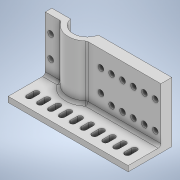
# Autodesk Inventor part: CLAMP2
Saved by Autodesk Inventor 2022 (Build 260153000, 153)
## iProperties
Created: 2022-02-10
Part Number: CLAMP2
Material: Generic
Document SubType Name: Modeling
Designer: 24sa01
Density: 1 g/cm^3
Appearance: Default
Author: 24sa01
Autodesk Inventor part; units mm, degrees
ref_plane "YZ Plane" through (0, 0, 0) normal (1, 0, 0) x (0, 1, 0)
ref_plane "XZ Plane" through (0, 0, 0) normal (0, 1, 0) x (-1, 0, 0)
ref_plane "XY Plane" through (0, 0, 0) normal (0, 0, 1) x (1, 0, 0)
sketch "Sketch1" plane through (0, 0, 0) normal (0, 1, 0) x (-1, 0, 0)
  line L0 (0, 0) -> (-139.7, 0)
  line L1 (-139.7, 0) -> (-139.7, -50.8)
  line L2 (-139.7, -50.8) -> (0, -50.8)
  line L3 (0, -50.8) -> (0, 0)
  line L4 (-12.7, -11.7475) -> (-12.7, -20.0025) construction
  line L5 (-15.875, -11.7475) -> (-15.875, -20.0025)
  line L6 (-9.525, -20.0025) -> (-9.525, -11.7475)
  arc A0 (-9.525, -11.7475) -> (-15.875, -11.7475) centre (-12.7, -11.7475) ccw
  arc A1 (-15.875, -20.0025) -> (-9.525, -20.0025) centre (-12.7, -20.0025) ccw
  line L7 (-25.4, -11.7475) -> (-25.4, -20.0025) construction
  line L8 (-28.575, -11.7475) -> (-28.575, -20.0025)
  line L9 (-22.225, -20.0025) -> (-22.225, -11.7475)
  arc A2 (-22.225, -11.7475) -> (-28.575, -11.7475) centre (-25.4, -11.7475) ccw
  arc A3 (-28.575, -20.0025) -> (-22.225, -20.0025) centre (-25.4, -20.0025) ccw
  line L10 (-50.8, -11.7475) -> (-50.8, -20.0025) construction
  line L11 (-47.625, -20.0025) -> (-47.625, -11.7475)
  line L12 (-53.975, -11.7475) -> (-53.975, -20.0025)
  arc A4 (-53.975, -20.0025) -> (-47.625, -20.0025) centre (-50.8, -20.0025) ccw
  arc A5 (-47.625, -11.7475) -> (-53.975, -11.7475) centre (-50.8, -11.7475) ccw
  line L13 (-41.275, -11.7475) -> (-41.275, -20.0025)
  line L14 (-38.1, -11.7475) -> (-38.1, -20.0025) construction
  arc A6 (-34.925, -11.7475) -> (-41.275, -11.7475) centre (-38.1, -11.7475) ccw
  arc A7 (-41.275, -20.0025) -> (-34.925, -20.0025) centre (-38.1, -20.0025) ccw
  line L15 (-34.925, -20.0025) -> (-34.925, -11.7475)
  line L16 (-76.2, -11.7475) -> (-76.2, -20.0025) construction
  line L17 (-73.025, -20.0025) -> (-73.025, -11.7475)
  line L18 (-79.375, -11.7475) -> (-79.375, -20.0025)
  arc A8 (-79.375, -20.0025) -> (-73.025, -20.0025) centre (-76.2, -20.0025) ccw
  arc A9 (-73.025, -11.7475) -> (-79.375, -11.7475) centre (-76.2, -11.7475) ccw
  line L19 (-66.675, -11.7475) -> (-66.675, -20.0025)
  line L20 (-63.5, -11.7475) -> (-63.5, -20.0025) construction
  arc A10 (-60.325, -11.7475) -> (-66.675, -11.7475) centre (-63.5, -11.7475) ccw
  arc A11 (-66.675, -20.0025) -> (-60.325, -20.0025) centre (-63.5, -20.0025) ccw
  line L21 (-60.325, -20.0025) -> (-60.325, -11.7475)
  line L22 (-101.6, -11.7475) -> (-101.6, -20.0025) construction
  line L23 (-98.425, -20.0025) -> (-98.425, -11.7475)
  line L24 (-104.775, -11.7475) -> (-104.775, -20.0025)
  arc A12 (-104.775, -20.0025) -> (-98.425, -20.0025) centre (-101.6, -20.0025) ccw
  arc A13 (-98.425, -11.7475) -> (-104.775, -11.7475) centre (-101.6, -11.7475) ccw
  line L25 (-92.075, -11.7475) -> (-92.075, -20.0025)
  line L26 (-88.9, -11.7475) -> (-88.9, -20.0025) construction
  arc A14 (-85.725, -11.7475) -> (-92.075, -11.7475) centre (-88.9, -11.7475) ccw
  arc A15 (-92.075, -20.0025) -> (-85.725, -20.0025) centre (-88.9, -20.0025) ccw
  line L27 (-85.725, -20.0025) -> (-85.725, -11.7475)
  line L28 (-127, -11.7475) -> (-127, -20.0025) construction
  line L29 (-123.825, -20.0025) -> (-123.825, -11.7475)
  line L30 (-130.175, -11.7475) -> (-130.175, -20.0025)
  arc A16 (-130.175, -20.0025) -> (-123.825, -20.0025) centre (-127, -20.0025) ccw
  arc A17 (-123.825, -11.7475) -> (-130.175, -11.7475) centre (-127, -11.7475) ccw
  line L31 (-117.475, -11.7475) -> (-117.475, -20.0025)
  line L32 (-114.3, -11.7475) -> (-114.3, -20.0025) construction
  arc A18 (-111.125, -11.7475) -> (-117.475, -11.7475) centre (-114.3, -11.7475) ccw
  arc A19 (-117.475, -20.0025) -> (-111.125, -20.0025) centre (-114.3, -20.0025) ccw
  line L33 (-111.125, -20.0025) -> (-111.125, -11.7475)
  point P0 (-12.7, -15.875)
  point P1 (-25.4, -15.875)
  point P2 (-50.8, -15.875)
  point P3 (-38.1, -15.875)
  point P4 (-76.2, -15.875)
  point P5 (-63.5, -15.875)
  point P6 (-101.6, -15.875)
  point P7 (-88.9, -15.875)
  point P8 (-127, -15.875)
  point P9 (-114.3, -15.875)
  dimension "d0" = 50.8
  dimension "d1" = 139.7
  dimension "d41" = 8.255
  dimension "d42" = 6.35
  dimension "d43" = 12.7
  dimension "d44" = 8.255
  dimension "d45" = 6.35
  dimension "d68" = 12.7
  dimension "d69" = 15.875
  dimension "d72" = 25.4
  constraints: 88 end point, 40 point on circle, 20 centre point, 8 tangent, 4 parallel, 2 horizontal, 2 midpoint, 2 vertical, 1 horizontal alignment, 1 perpendicular, 96 other
  measures "d0" distance of L0.end L1.end
  measures "d1" distance of L1.end L2.end
  measures "d41" distance of L4.start L4.end
  measures "d42" diameter of A1
  measures "d43" distance from line of L3 point (-12.7, -15.875)
  measures "d44" distance of L7.start L7.end
  measures "d45" diameter of A3
  measures "d68" distance of point (-25.4, -15.875) point (-12.7, -15.875)
  measures "d69" distance from line of point (-12.7, -15.875) L0
  measures "d72" distance of point (-25.4, -15.875) point (-50.8, -15.875)
extrude "Extrusion1" add sketch "Sketch1" along normal blind 6.35
sketch "Sketch2" plane through (0, 6.35, 0) normal (0, 1, 0) x (1, 0, 0)
  line L0 (139.7, 50.8) -> (0, 50.8)
  circle A0 centre (38.1, 53.975) radius 16.51
  line L1 (0, 50.8) -> (0, 0) projected
  circle A1 centre (38.1, 53.975) radius 22.225
  line L2 (18.6727, 43.18) -> (0, 43.18)
  line L3 (139.7, 50.8) -> (0, 50.8) projected
  line L4 (53.6543, 38.1) -> (139.7, 38.1)
  line L5 (139.7, 0) -> (139.7, 50.8) projected
  point P0 (54.3018, 50.8)
  point P1 (21.8982, 50.8)
  dimension "d22" = 33.02
  dimension "d23" = 3.175
  dimension "d24" = 38.1
  dimension "d25" = 44.45
  dimension "d26" = 7.62
  dimension "d27" = 12.7
  constraints: 6 end point, 2 centre point, 2 point on circle, 2 point on line, 1 coincident, 1 horizontal, 1 perpendicular
  measures "d22" diameter of A0
  measures "d23" distance from line of L0 A0.centre
  measures "d24" distance from line of L1 A0.centre
  measures "d25" diameter of A1
  measures "d26" distance between parallel lines of L0 L2
  measures "d27" distance between parallel lines of L0 L4
extrude "Extrusion2" add sketch "Sketch2" along normal blind 63.5 contours L5 L4 A1 L0 | A1 L0 A0 | L2 L1 L0 A1 picked at (21.7662, 42.0556)
sketch "Sketch3" plane through (0, 6.35, -43.18) normal (0, 0, 1) x (1, 0, 0)
  line L0 (139.7, 0) -> (139.7, 63.5) projected
  line L1 (0, 0) -> (0, 63.5) projected
  line L2 (0, 63.5) -> (18.6727, 63.5) projected
  line L3 (53.6543, 63.5) -> (139.7, 63.5) projected
  line L4 (54.3018, 0) -> (21.8982, 0) projected
  point P0 (0, -6.35)
  point P1 (6.35, 44.45)
  point P2 (69.85, 44.45)
  point P3 (6.35, 19.05)
  point P4 (69.85, 19.05)
  dimension "d30" = 69.85
  dimension "d31" = 6.35
  dimension "d32" = 19.05
  dimension "d33" = 19.05
  dimension "d52" = 6.35
  dimension "d53" = 69.85
  dimension "d54" = 19.05
  dimension "d55" = 19.05
  measures "d30" distance from line of L0 point (69.85, 44.45)
  measures "d31" distance from line of L1 point (6.35, 44.45)
  measures "d32" distance from line of L2 point (6.35, 44.45)
  measures "d33" distance from line of L3 point (69.85, 44.45)
  measures "d52" distance from line of L1 point (6.35, 19.05)
  measures "d53" distance from line of L0 point (69.85, 19.05)
  measures "d54" distance from line of L4 point (69.85, 19.05)
  measures "d55" distance from line of L4 point (6.35, 19.05)
hole "Hole1" at (6.35, 50.8, -43.18) at (6.35, 25.4, -43.18) at (69.85, 25.4, -43.18) at (69.85, 50.8, -43.18) direction (0, 0, -1) diameter 6.7564 end through all start extended yes
fillet "Fillet1" radius 3.175 2 edges at (18.6727, 38.1, -43.18) (53.6543, 38.1, -38.1)
sketch "Sketch6" plane through (0, 6.35, 0) normal (0, 1, 0) x (1, 0, 0)
  circle A0 centre (38.1, 53.975) radius 16.51
  arc A1 (21.8982, 50.8) -> (54.3018, 50.8) centre (38.1, 53.975) ccw projected
  point P0 (0, 0)
  point P1 (19.2581, 43.18)
  point P2 (44.2419, 43.18)
  dimension "d49" = 33.02
  constraints: 3 other
extrude "Extrusion3" cut sketch "Sketch6" against normal blind 25.4
sketch "Sketch7" plane through (139.7, 6.35, -38.1) normal (0, 0, 1) x (1, 0, 0)
  point P0 (-139.7, -6.35)
  point P1 (-44.6065, 44.5733)
  point P2 (-19.2065, 44.5733)
  point P3 (-44.6065, 12.8233)
  point P4 (-19.2065, 12.8233)
  point P5 (-57.3065, 44.5733)
  point P6 (-31.9065, 44.5733)
  point P7 (-57.3065, 12.8233)
  point P8 (-31.9065, 12.8233)
  point P9 (-6.5065, 44.5733)
  point P10 (-6.5065, 12.8233)
  dimension "d63" = 25.4
  dimension "d64" = 31.75
  dimension "d65" = 12.7
  dimension "d66" = 12.7
  dimension "d67" = 12.7
  constraints: 5 vertical alignment, 4 horizontal alignment
  measures "d63" distance of point (-19.206, 44.573) point (-44.606, 44.573)
  measures "d64" distance of point (-19.206, 12.823) point (-19.206, 44.573)
  measures "d65" distance of point (-44.606, 44.573) point (-57.306, 44.573)
  measures "d66" distance of point (-31.906, 44.573) point (-44.606, 44.573)
  measures "d67" distance of point (-6.506, 44.573) point (-19.206, 44.573)
hole "Hole2" at (95.0935, 50.9233, -38.1) at (120.4935, 50.9233, -38.1) at (95.0935, 19.1733, -38.1) at (120.4935, 19.1733, -38.1) at (82.3935, 50.9233, -38.1) at (107.7935, 50.9233, -38.1) at (82.3935, 19.1733, -38.1) at (107.7935, 19.1733, -38.1) at (133.1935, 50.9233, -38.1) at (133.1935, 19.1733, -38.1) direction (0, 0, -1) diameter 6.7564 end through all
fillet "Fillet2" radius 3.175 5 edges at (53.778, 6.35, -37.8949) (35.1561, 6.35, -31.9458) (18.3929, 6.35, -42.8001) (8.4434, 6.35, -43.18) (97.3003, 6.35, -38.1)
body "Solid1"
